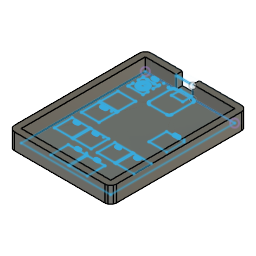
case housing (Autodesk Fusion 360 design; units mm, degrees)
part number: 2026-08-13-11-53-39-217
Autodesk Fusion 360 part; units mm, degrees
(part 1 of 10)
sketch "controller-Edge_Cuts" plane through (0, 0, 3) normal (0, 0, 1) x (1, 0, 0)
  line L0 (34.5096, 49.5231) -> (34.5231, 49.5096)
  line L1 (34.5231, 49.5096) -> (34.525, 49.5)
  line L2 (34.525, 49.5) -> (34.525, -49)
  line L3 (34.525, -49) -> (34.5231, -49.0096)
  line L4 (34.5231, -49.0096) -> (34.5096, -49.0231)
  line L5 (34.5096, -49.0231) -> (34.5, -49.025)
  line L6 (34.5, -49.025) -> (-36.5, -49.025)
  line L7 (-36.5, -49.025) -> (-36.5096, -49.0231)
  line L8 (-36.5096, -49.0231) -> (-36.5231, -49.0096)
  line L9 (-36.5231, -49.0096) -> (-36.525, -49)
  line L10 (-36.525, -49) -> (-36.525, 49.5)
  line L11 (-36.525, 49.5) -> (-36.5231, 49.5096)
  line L12 (-36.5231, 49.5096) -> (-36.5096, 49.5231)
  line L13 (-36.5096, 49.5231) -> (-36.5, 49.525)
  line L14 (-36.5, 49.525) -> (34.5, 49.525)
  line L15 (34.5, 49.525) -> (34.5096, 49.5231)
  line L16 (-36.475, 49.475) -> (-36.475, -48.975)
  line L17 (-36.475, -48.975) -> (34.475, -48.975)
  line L18 (34.475, -48.975) -> (34.475, 49.475)
  line L19 (34.475, 49.475) -> (-36.475, 49.475)
  line L20 (-41.1311, 51.9726) -> (-38.9726, 54.1311)
  line L21 (-38.9726, 54.1311) -> (-36.9925, 54.525)
  line L22 (-36.9925, 54.525) -> (34.9925, 54.525)
  line L23 (34.9925, 54.525) -> (36.9726, 54.1311)
  line L24 (36.9726, 54.1311) -> (39.1311, 51.9726)
  line L25 (39.1311, 51.9726) -> (39.525, 49.9925)
  line L26 (39.525, 49.9925) -> (39.525, -49.4925)
  line L27 (39.525, -49.4925) -> (39.1311, -51.4726)
  line L28 (39.1311, -51.4726) -> (36.9726, -53.6311)
  line L29 (36.9726, -53.6311) -> (34.9925, -54.025)
  line L30 (34.9925, -54.025) -> (-36.9925, -54.025)
  line L31 (-36.9925, -54.025) -> (-38.9726, -53.6311)
  line L32 (-38.9726, -53.6311) -> (-41.1311, -51.4726)
  line L33 (-41.1311, -51.4726) -> (-41.525, -49.4925)
  line L34 (-41.525, -49.4925) -> (-41.525, 49.9925)
  line L35 (-41.525, 49.9925) -> (-41.1311, 51.9726)
  dimension "d53" = -5
extrude "Extrude15" add sketch "controller-Edge_Cuts" along normal blind 3 contours L16 L17 L18 L19 makes body 1
extrude "Extrude16" add sketch "controller-Edge_Cuts" along normal blind 13 separate body contours L20 L21 L22 L23 L24 L25 L26 L27 L28 L29 L30 L31 L32 L33 L34 L35 makes body 2
sketch "controller-F_Silkscreen" plane through (0, 0, 6) normal (0, 0, 1) x (1, 0, 0)
  line L0 (-2.662, -31.4596) -> (-2.6296, -31.492)
  line L1 (-2.6296, -31.492) -> (-2.625, -31.515)
  line L2 (-2.625, -31.515) -> (-2.625, -45.485)
  line L3 (-2.625, -45.485) -> (-2.6296, -45.508)
  line L4 (-2.6296, -45.508) -> (-2.662, -45.5404)
  line L5 (-2.662, -45.5404) -> (-2.685, -45.545)
  line L6 (-2.685, -45.545) -> (-16.655, -45.545)
  line L7 (-16.655, -45.545) -> (-16.678, -45.5404)
  line L8 (-16.678, -45.5404) -> (-16.7104, -45.508)
  line L9 (-16.7104, -45.508) -> (-16.715, -45.485)
  line L10 (-16.715, -45.485) -> (-16.715, -31.515)
  line L11 (-16.715, -31.515) -> (-16.7104, -31.492)
  line L12 (-16.7104, -31.492) -> (-16.678, -31.4596)
  line L13 (-16.678, -31.4596) -> (-16.655, -31.455)
  line L14 (-16.655, -31.455) -> (-2.685, -31.455)
  line L15 (-2.685, -31.455) -> (-2.662, -31.4596)
  line L16 (-16.595, -31.575) -> (-16.595, -45.425)
  line L17 (-16.595, -45.425) -> (-2.745, -45.425)
  line L18 (-2.745, -45.425) -> (-2.745, -31.575)
  line L19 (-2.745, -31.575) -> (-16.595, -31.575)
  line L20 (12.428, -31.4596) -> (12.4604, -31.492)
  line L21 (12.4604, -31.492) -> (12.465, -31.515)
  line L22 (12.465, -31.515) -> (12.465, -45.485)
  line L23 (12.465, -45.485) -> (12.4604, -45.508)
  line L24 (12.4604, -45.508) -> (12.428, -45.5404)
  line L25 (12.428, -45.5404) -> (12.405, -45.545)
  line L26 (12.405, -45.545) -> (-1.565, -45.545)
  line L27 (-1.565, -45.545) -> (-1.588, -45.5404)
  line L28 (-1.588, -45.5404) -> (-1.6204, -45.508)
  line L29 (-1.6204, -45.508) -> (-1.625, -45.485)
  line L30 (-1.625, -45.485) -> (-1.625, -31.515)
  line L31 (-1.625, -31.515) -> (-1.6204, -31.492)
  line L32 (-1.6204, -31.492) -> (-1.588, -31.4596)
  line L33 (-1.588, -31.4596) -> (-1.565, -31.455)
  line L34 (-1.565, -31.455) -> (12.405, -31.455)
  line L35 (12.405, -31.455) -> (12.428, -31.4596)
  line L36 (-1.505, -31.575) -> (-1.505, -45.425)
  line L37 (-1.505, -45.425) -> (12.345, -45.425)
  line L38 (12.345, -45.425) -> (12.345, -31.575)
  line L39 (12.345, -31.575) -> (-1.505, -31.575)
  line L40 (-10.5674, -30.0065) -> (-10.5654, -30.0064)
  line L41 (-10.5654, -30.0064) -> (-10.5628, -30.007)
  line L42 (-10.5628, -30.007) -> (-10.5601, -30.0073)
  line L43 (-10.5601, -30.0073) -> (-10.5583, -30.008)
  line L44 (-10.5583, -30.008) -> (-10.551, -30.0097)
  line L45 (-10.551, -30.0097) -> (-10.4082, -30.0573)
  line L46 (-10.4082, -30.0573) -> (-10.3948, -30.0633)
  line L47 (-10.3948, -30.0633) -> (-10.3727, -30.0825)
  line L48 (-10.3727, -30.0825) -> (-10.3596, -30.1086)
  line L49 (-10.3596, -30.1086) -> (-10.3575, -30.1378)
  line L50 (-10.3575, -30.1378) -> (-10.3667, -30.1656)
  line L51 (-10.3667, -30.1656) -> (-10.3859, -30.1877)
  line L52 (-10.3859, -30.1877) -> (-10.4121, -30.2008)
  line L53 (-10.4121, -30.2008) -> (-10.4413, -30.2028)
  line L54 (-10.4413, -30.2028) -> (-10.4556, -30.1996)
  line L55 (-10.4556, -30.1996) -> (-10.5869, -30.1558)
  line L56 (-10.5869, -30.1558) -> (-10.7952, -30.1558)
  line L57 (-10.7952, -30.1558) -> (-10.8637, -30.1901)
  line L58 (-10.8637, -30.1901) -> (-10.8941, -30.2205)
  line L59 (-10.8941, -30.2205) -> (-10.9283, -30.289)
  line L60 (-10.9283, -30.289) -> (-10.9283, -30.3488)
  line L61 (-10.9283, -30.3488) -> (-10.8941, -30.4173)
  line L62 (-10.8941, -30.4173) -> (-10.8637, -30.4478)
  line L63 (-10.8637, -30.4478) -> (-10.7867, -30.4862)
  line L64 (-10.7867, -30.4862) -> (-10.6042, -30.5319)
  line L65 (-10.6042, -30.5319) -> (-10.6031, -30.5323)
  line L66 (-10.6031, -30.5323) -> (-10.6026, -30.5323)
  line L67 (-10.6026, -30.5323) -> (-10.5965, -30.5346)
  line L68 (-10.5965, -30.5346) -> (-10.5903, -30.5368)
  line L69 (-10.5903, -30.5368) -> (-10.5899, -30.5371)
  line L70 (-10.5899, -30.5371) -> (-10.5888, -30.5375)
  line L71 (-10.5888, -30.5375) -> (-10.4936, -30.5852)
  line L72 (-10.4936, -30.5852) -> (-10.4873, -30.5891)
  line L73 (-10.4873, -30.5891) -> (-10.4855, -30.5899)
  line L74 (-10.4855, -30.5899) -> (-10.4834, -30.5916)
  line L75 (-10.4834, -30.5916) -> (-10.4812, -30.593)
  line L76 (-10.4812, -30.593) -> (-10.4799, -30.5945)
  line L77 (-10.4799, -30.5945) -> (-10.4741, -30.5992)
  line L78 (-10.4741, -30.5992) -> (-10.4265, -30.6468)
  line L79 (-10.4265, -30.6468) -> (-10.4218, -30.6526)
  line L80 (-10.4218, -30.6526) -> (-10.4203, -30.6539)
  line L81 (-10.4203, -30.6539) -> (-10.4189, -30.6561)
  line L82 (-10.4189, -30.6561) -> (-10.4172, -30.6582)
  line L83 (-10.4172, -30.6582) -> (-10.4164, -30.66)
  line L84 (-10.4164, -30.66) -> (-10.4124, -30.6663)
  line L85 (-10.4124, -30.6663) -> (-10.3648, -30.7616)
  line L86 (-10.3648, -30.7616) -> (-10.3596, -30.7753)
  line L87 (-10.3596, -30.7753) -> (-10.3594, -30.778)
  line L88 (-10.3594, -30.778) -> (-10.3583, -30.7805)
  line L89 (-10.3583, -30.7805) -> (-10.3569, -30.7951)
  line L90 (-10.3569, -30.7951) -> (-10.3569, -30.8903)
  line L91 (-10.3569, -30.8903) -> (-10.3583, -30.905)
  line L92 (-10.3583, -30.905) -> (-10.3594, -30.9075)
  line L93 (-10.3594, -30.9075) -> (-10.3596, -30.9102)
  line L94 (-10.3596, -30.9102) -> (-10.3648, -30.9239)
  line L95 (-10.3648, -30.9239) -> (-10.4124, -31.0191)
  line L96 (-10.4124, -31.0191) -> (-10.4164, -31.0254)
  line L97 (-10.4164, -31.0254) -> (-10.4172, -31.0272)
  line L98 (-10.4172, -31.0272) -> (-10.4189, -31.0293)
  line L99 (-10.4189, -31.0293) -> (-10.4203, -31.0316)
  line L100 (-10.4203, -31.0316) -> (-10.4218, -31.0329)
  line L101 (-10.4218, -31.0329) -> (-10.4265, -31.0386)
  line L102 (-10.4265, -31.0386) -> (-10.4741, -31.0862)
  line L103 (-10.4741, -31.0862) -> (-10.4799, -31.0909)
  line L104 (-10.4799, -31.0909) -> (-10.4812, -31.0924)
  line L105 (-10.4812, -31.0924) -> (-10.4834, -31.0939)
  line L106 (-10.4834, -31.0939) -> (-10.4855, -31.0956)
  line L107 (-10.4855, -31.0956) -> (-10.4873, -31.0963)
  line L108 (-10.4873, -31.0963) -> (-10.4936, -31.1003)
  line L109 (-10.4936, -31.1003) -> (-10.5888, -31.1479)
  line L110 (-10.5888, -31.1479) -> (-10.6026, -31.1532)
  line L111 (-10.6026, -31.1532) -> (-10.6053, -31.1533)
  line L112 (-10.6053, -31.1533) -> (-10.6077, -31.1544)
  line L113 (-10.6077, -31.1544) -> (-10.6224, -31.1558)
  line L114 (-10.6224, -31.1558) -> (-10.8605, -31.1558)
  line L115 (-10.8605, -31.1558) -> (-10.8679, -31.1551)
  line L116 (-10.8679, -31.1551) -> (-10.8699, -31.1552)
  line L117 (-10.8699, -31.1552) -> (-10.8725, -31.1546)
  line L118 (-10.8725, -31.1546) -> (-10.8751, -31.1544)
  line L119 (-10.8751, -31.1544) -> (-10.8769, -31.1536)
  line L120 (-10.8769, -31.1536) -> (-10.8842, -31.152)
  line L121 (-10.8842, -31.152) -> (-11.0271, -31.1044)
  line L122 (-11.0271, -31.1044) -> (-11.0405, -31.0984)
  line L123 (-11.0405, -31.0984) -> (-11.0626, -31.0792)
  line L124 (-11.0626, -31.0792) -> (-11.0757, -31.053)
  line L125 (-11.0757, -31.053) -> (-11.0777, -31.0238)
  line L126 (-11.0777, -31.0238) -> (-11.0685, -30.9961)
  line L127 (-11.0685, -30.9961) -> (-11.0493, -30.974)
  line L128 (-11.0493, -30.974) -> (-11.0231, -30.9609)
  line L129 (-11.0231, -30.9609) -> (-10.994, -30.9588)
  line L130 (-10.994, -30.9588) -> (-10.9796, -30.962)
  line L131 (-10.9796, -30.962) -> (-10.8483, -31.0058)
  line L132 (-10.8483, -31.0058) -> (-10.6401, -31.0058)
  line L133 (-10.6401, -31.0058) -> (-10.5716, -30.9716)
  line L134 (-10.5716, -30.9716) -> (-10.5412, -30.9412)
  line L135 (-10.5412, -30.9412) -> (-10.5069, -30.8726)
  line L136 (-10.5069, -30.8726) -> (-10.5069, -30.8128)
  line L137 (-10.5069, -30.8128) -> (-10.5412, -30.7443)
  line L138 (-10.5412, -30.7443) -> (-10.5716, -30.7139)
  line L139 (-10.5716, -30.7139) -> (-10.6486, -30.6754)
  line L140 (-10.6486, -30.6754) -> (-10.831, -30.6298)
  line L141 (-10.831, -30.6298) -> (-10.8321, -30.6294)
  line L142 (-10.8321, -30.6294) -> (-10.8327, -30.6293)
  line L143 (-10.8327, -30.6293) -> (-10.8388, -30.627)
  line L144 (-10.8388, -30.627) -> (-10.8449, -30.6248)
  line L145 (-10.8449, -30.6248) -> (-10.8453, -30.6245)
  line L146 (-10.8453, -30.6245) -> (-10.8464, -30.6241)
  line L147 (-10.8464, -30.6241) -> (-10.9416, -30.5765)
  line L148 (-10.9416, -30.5765) -> (-10.9479, -30.5725)
  line L149 (-10.9479, -30.5725) -> (-10.9498, -30.5717)
  line L150 (-10.9498, -30.5717) -> (-10.9518, -30.5701)
  line L151 (-10.9518, -30.5701) -> (-10.9541, -30.5686)
  line L152 (-10.9541, -30.5686) -> (-10.9554, -30.5671)
  line L153 (-10.9554, -30.5671) -> (-10.9611, -30.5624)
  line L154 (-10.9611, -30.5624) -> (-11.0087, -30.5148)
  line L155 (-11.0087, -30.5148) -> (-11.0135, -30.5091)
  line L156 (-11.0135, -30.5091) -> (-11.015, -30.5078)
  line L157 (-11.015, -30.5078) -> (-11.0164, -30.5055)
  line L158 (-11.0164, -30.5055) -> (-11.0181, -30.5034)
  line L159 (-11.0181, -30.5034) -> (-11.0188, -30.5016)
  line L160 (-11.0188, -30.5016) -> (-11.0228, -30.4953)
  line L161 (-11.0228, -30.4953) -> (-11.0704, -30.4001)
  line L162 (-11.0704, -30.4001) -> (-11.0757, -30.3863)
  line L163 (-11.0757, -30.3863) -> (-11.0759, -30.3837)
  line L164 (-11.0759, -30.3837) -> (-11.0769, -30.3812)
  line L165 (-11.0769, -30.3812) -> (-11.0783, -30.3665)
  line L166 (-11.0783, -30.3665) -> (-11.0783, -30.2713)
  line L167 (-11.0783, -30.2713) -> (-11.0769, -30.2567)
  line L168 (-11.0769, -30.2567) -> (-11.0759, -30.2542)
  line L169 (-11.0759, -30.2542) -> (-11.0757, -30.2515)
  line L170 (-11.0757, -30.2515) -> (-11.0704, -30.2378)
  line L171 (-11.0704, -30.2378) -> (-11.0228, -30.1425)
  line L172 (-11.0228, -30.1425) -> (-11.0188, -30.1362)
  line L173 (-11.0188, -30.1362) -> (-11.0181, -30.1344)
  line L174 (-11.0181, -30.1344) -> (-11.0164, -30.1323)
  line L175 (-11.0164, -30.1323) -> (-11.015, -30.1301)
  line L176 (-11.015, -30.1301) -> (-11.0135, -30.1288)
  line L177 (-11.0135, -30.1288) -> (-11.0087, -30.123)
  line L178 (-11.0087, -30.123) -> (-10.9611, -30.0754)
  line L179 (-10.9611, -30.0754) -> (-10.9554, -30.0707)
  line L180 (-10.9554, -30.0707) -> (-10.9541, -30.0692)
  line L181 (-10.9541, -30.0692) -> (-10.9518, -30.0678)
  line L182 (-10.9518, -30.0678) -> (-10.9498, -30.0661)
  line L183 (-10.9498, -30.0661) -> (-10.9479, -30.0653)
  line L184 (-10.9479, -30.0653) -> (-10.9416, -30.0614)
  line L185 (-10.9416, -30.0614) -> (-10.8464, -30.0137)
  line L186 (-10.8464, -30.0137) -> (-10.8327, -30.0085)
  line L187 (-10.8327, -30.0085) -> (-10.83, -30.0083)
  line L188 (-10.83, -30.0083) -> (-10.8275, -30.0073)
  line L189 (-10.8275, -30.0073) -> (-10.8129, -30.0058)
  line L190 (-10.8129, -30.0058) -> (-10.5748, -30.0058)
  line L191 (-10.5748, -30.0058) -> (-10.5674, -30.0065)
  line L192 (-8.6152, -30.0073) -> (-8.6077, -30.0073)
  line L193 (-8.6077, -30.0073) -> (-8.601, -30.0101)
  line L194 (-8.601, -30.0101) -> (-8.5938, -30.0115)
  line L195 (-8.5938, -30.0115) -> (-8.5876, -30.0156)
  line L196 (-8.5876, -30.0156) -> (-8.5807, -30.0185)
  line L197 (-8.5807, -30.0185) -> (-8.5755, -30.0237)
  line L198 (-8.5755, -30.0237) -> (-8.5694, -30.0277)
  line L199 (-8.5694, -30.0277) -> (-8.5653, -30.0339)
  line L200 (-8.5653, -30.0339) -> (-8.56, -30.0392)
  line L201 (-8.56, -30.0392) -> (-8.5572, -30.0459)
  line L202 (-8.5572, -30.0459) -> (-8.5531, -30.052)
  line L203 (-8.5531, -30.052) -> (-8.5517, -30.0593)
  line L204 (-8.5517, -30.0593) -> (-8.5488, -30.0662)
  line L205 (-8.5488, -30.0662) -> (-8.5474, -30.0807)
  line L206 (-8.5474, -30.0807) -> (-8.5474, -30.0807)
  line L207 (-8.5474, -30.0807) -> (-8.5474, -30.0808)
  line L208 (-8.5474, -30.0808) -> (-8.5474, -30.0808)
  line L209 (-8.5474, -30.0808) -> (-8.5474, -31.0058)
  line L210 (-8.5474, -31.0058) -> (-8.3367, -31.0058)
  line L211 (-8.3367, -31.0058) -> (-8.322, -31.0073)
  line L212 (-8.322, -31.0073) -> (-8.295, -31.0185)
  line L213 (-8.295, -31.0185) -> (-8.2743, -31.0392)
  line L214 (-8.2743, -31.0392) -> (-8.2631, -31.0662)
  line L215 (-8.2631, -31.0662) -> (-8.2631, -31.0955)
  line L216 (-8.2631, -31.0955) -> (-8.2743, -31.1225)
  line L217 (-8.2743, -31.1225) -> (-8.295, -31.1432)
  line L218 (-8.295, -31.1432) -> (-8.322, -31.1544)
  line L219 (-8.322, -31.1544) -> (-8.3367, -31.1558)
  line L220 (-8.3367, -31.1558) -> (-8.9081, -31.1558)
  line L221 (-8.9081, -31.1558) -> (-8.9227, -31.1544)
  line L222 (-8.9227, -31.1544) -> (-8.9498, -31.1432)
  line L223 (-8.9498, -31.1432) -> (-8.9705, -31.1225)
  line L224 (-8.9705, -31.1225) -> (-8.9817, -31.0955)
  line L225 (-8.9817, -31.0955) -> (-8.9817, -31.0662)
  line L226 (-8.9817, -31.0662) -> (-8.9705, -31.0392)
  line L227 (-8.9705, -31.0392) -> (-8.9498, -31.0185)
  line L228 (-8.9498, -31.0185) -> (-8.9227, -31.0073)
  line L229 (-8.9227, -31.0073) -> (-8.9081, -31.0058)
  line L230 (-8.9081, -31.0058) -> (-8.6974, -31.0058)
  line L231 (-8.6974, -31.0058) -> (-8.6974, -30.3095)
  line L232 (-8.6974, -30.3095) -> (-8.7598, -30.3719)
  line L233 (-8.7598, -30.3719) -> (-8.7656, -30.3767)
  line L234 (-8.7656, -30.3767) -> (-8.7669, -30.3782)
  line L235 (-8.7669, -30.3782) -> (-8.7691, -30.3796)
  line L236 (-8.7691, -30.3796) -> (-8.7712, -30.3813)
  line L237 (-8.7712, -30.3813) -> (-8.773, -30.382)
  line L238 (-8.773, -30.382) -> (-8.7793, -30.386)
  line L239 (-8.7793, -30.386) -> (-8.8746, -30.4336)
  line L240 (-8.8746, -30.4336) -> (-8.8883, -30.4389)
  line L241 (-8.8883, -30.4389) -> (-8.9175, -30.4409)
  line L242 (-8.9175, -30.4409) -> (-8.9452, -30.4317)
  line L243 (-8.9452, -30.4317) -> (-8.9673, -30.4125)
  line L244 (-8.9673, -30.4125) -> (-8.9804, -30.3863)
  line L245 (-8.9804, -30.3863) -> (-8.9825, -30.3572)
  line L246 (-8.9825, -30.3572) -> (-8.9733, -30.3294)
  line L247 (-8.9733, -30.3294) -> (-8.9541, -30.3073)
  line L248 (-8.9541, -30.3073) -> (-8.9416, -30.2995)
  line L249 (-8.9416, -30.2995) -> (-8.8573, -30.2573)
  line L250 (-8.8573, -30.2573) -> (-8.7759, -30.1759)
  line L251 (-8.7759, -30.1759) -> (-8.6848, -30.0392)
  line L252 (-8.6848, -30.0392) -> (-8.6848, -30.0392)
  line L253 (-8.6848, -30.0392) -> (-8.6847, -30.0392)
  line L254 (-8.6847, -30.0392) -> (-8.6847, -30.0391)
  line L255 (-8.6847, -30.0391) -> (-8.6755, -30.0278)
  line L256 (-8.6755, -30.0278) -> (-8.6693, -30.0237)
  line L257 (-8.6693, -30.0237) -> (-8.664, -30.0185)
  line L258 (-8.664, -30.0185) -> (-8.6573, -30.0156)
  line L259 (-8.6573, -30.0156) -> (-8.6512, -30.0116)
  line L260 (-8.6512, -30.0116) -> (-8.6439, -30.0101)
  line L261 (-8.6439, -30.0101) -> (-8.637, -30.0073)
  line L262 (-8.637, -30.0073) -> (-8.6297, -30.0073)
  line L263 (-8.6297, -30.0073) -> (-8.6225, -30.0058)
  line L264 (-8.6225, -30.0058) -> (-8.6152, -30.0073)
  line L265 (4.5226, -30.0065) -> (4.5246, -30.0064)
  line L266 (4.5246, -30.0064) -> (4.5272, -30.007)
  line L267 (4.5272, -30.007) -> (4.5299, -30.0073)
  line L268 (4.5299, -30.0073) -> (4.5317, -30.008)
  line L269 (4.5317, -30.008) -> (4.539, -30.0097)
  line L270 (4.539, -30.0097) -> (4.6818, -30.0573)
  line L271 (4.6818, -30.0573) -> (4.6952, -30.0633)
  line L272 (4.6952, -30.0633) -> (4.7173, -30.0825)
  line L273 (4.7173, -30.0825) -> (4.7304, -30.1086)
  line L274 (4.7304, -30.1086) -> (4.7325, -30.1378)
  line L275 (4.7325, -30.1378) -> (4.7233, -30.1656)
  line L276 (4.7233, -30.1656) -> (4.7041, -30.1877)
  line L277 (4.7041, -30.1877) -> (4.6779, -30.2008)
  line L278 (4.6779, -30.2008) -> (4.6487, -30.2028)
  line L279 (4.6487, -30.2028) -> (4.6344, -30.1996)
  line L280 (4.6344, -30.1996) -> (4.5031, -30.1558)
  line L281 (4.5031, -30.1558) -> (4.2948, -30.1558)
  line L282 (4.2948, -30.1558) -> (4.2263, -30.1901)
  line L283 (4.2263, -30.1901) -> (4.1959, -30.2205)
  line L284 (4.1959, -30.2205) -> (4.1617, -30.289)
  line L285 (4.1617, -30.289) -> (4.1617, -30.3488)
  line L286 (4.1617, -30.3488) -> (4.1959, -30.4173)
  line L287 (4.1959, -30.4173) -> (4.2263, -30.4478)
  line L288 (4.2263, -30.4478) -> (4.3033, -30.4862)
  line L289 (4.3033, -30.4862) -> (4.4858, -30.5319)
  line L290 (4.4858, -30.5319) -> (4.4869, -30.5323)
  line L291 (4.4869, -30.5323) -> (4.4874, -30.5323)
  line L292 (4.4874, -30.5323) -> (4.4935, -30.5346)
  line L293 (4.4935, -30.5346) -> (4.4997, -30.5368)
  line L294 (4.4997, -30.5368) -> (4.5001, -30.5371)
  line L295 (4.5001, -30.5371) -> (4.5012, -30.5375)
  line L296 (4.5012, -30.5375) -> (4.5964, -30.5852)
  line L297 (4.5964, -30.5852) -> (4.6027, -30.5891)
  line L298 (4.6027, -30.5891) -> (4.6045, -30.5899)
  line L299 (4.6045, -30.5899) -> (4.6066, -30.5916)
  line L300 (4.6066, -30.5916) -> (4.6088, -30.593)
  line L301 (4.6088, -30.593) -> (4.6101, -30.5945)
  line L302 (4.6101, -30.5945) -> (4.6159, -30.5992)
  line L303 (4.6159, -30.5992) -> (4.6635, -30.6468)
  line L304 (4.6635, -30.6468) -> (4.6682, -30.6526)
  line L305 (4.6682, -30.6526) -> (4.6697, -30.6539)
  line L306 (4.6697, -30.6539) -> (4.6711, -30.6561)
  line L307 (4.6711, -30.6561) -> (4.6728, -30.6582)
  line L308 (4.6728, -30.6582) -> (4.6736, -30.66)
  line L309 (4.6736, -30.66) -> (4.6776, -30.6663)
  line L310 (4.6776, -30.6663) -> (4.7252, -30.7616)
  line L311 (4.7252, -30.7616) -> (4.7304, -30.7753)
  line L312 (4.7304, -30.7753) -> (4.7306, -30.778)
  line L313 (4.7306, -30.778) -> (4.7317, -30.7805)
  line L314 (4.7317, -30.7805) -> (4.7331, -30.7951)
  line L315 (4.7331, -30.7951) -> (4.7331, -30.8903)
  line L316 (4.7331, -30.8903) -> (4.7317, -30.905)
  line L317 (4.7317, -30.905) -> (4.7306, -30.9075)
  line L318 (4.7306, -30.9075) -> (4.7304, -30.9102)
  line L319 (4.7304, -30.9102) -> (4.7252, -30.9239)
  line L320 (4.7252, -30.9239) -> (4.6776, -31.0191)
  line L321 (4.6776, -31.0191) -> (4.6736, -31.0254)
  line L322 (4.6736, -31.0254) -> (4.6728, -31.0272)
  line L323 (4.6728, -31.0272) -> (4.6711, -31.0293)
  line L324 (4.6711, -31.0293) -> (4.6697, -31.0316)
  line L325 (4.6697, -31.0316) -> (4.6682, -31.0329)
  line L326 (4.6682, -31.0329) -> (4.6635, -31.0386)
  line L327 (4.6635, -31.0386) -> (4.6159, -31.0862)
  line L328 (4.6159, -31.0862) -> (4.6101, -31.0909)
  line L329 (4.6101, -31.0909) -> (4.6088, -31.0924)
  line L330 (4.6088, -31.0924) -> (4.6066, -31.0939)
  line L331 (4.6066, -31.0939) -> (4.6045, -31.0956)
  line L332 (4.6045, -31.0956) -> (4.6027, -31.0963)
  line L333 (4.6027, -31.0963) -> (4.5964, -31.1003)
  line L334 (4.5964, -31.1003) -> (4.5012, -31.1479)
  line L335 (4.5012, -31.1479) -> (4.4874, -31.1532)
  line L336 (4.4874, -31.1532) -> (4.4847, -31.1533)
  line L337 (4.4847, -31.1533) -> (4.4823, -31.1544)
  line L338 (4.4823, -31.1544) -> (4.4676, -31.1558)
  line L339 (4.4676, -31.1558) -> (4.2295, -31.1558)
  line L340 (4.2295, -31.1558) -> (4.2221, -31.1551)
  line L341 (4.2221, -31.1551) -> (4.2201, -31.1552)
  line L342 (4.2201, -31.1552) -> (4.2175, -31.1546)
  line L343 (4.2175, -31.1546) -> (4.2149, -31.1544)
  line L344 (4.2149, -31.1544) -> (4.2131, -31.1536)
  line L345 (4.2131, -31.1536) -> (4.2058, -31.152)
  line L346 (4.2058, -31.152) -> (4.063, -31.1044)
  line L347 (4.063, -31.1044) -> (4.0495, -31.0984)
  line L348 (4.0495, -31.0984) -> (4.0274, -31.0792)
  line L349 (4.0274, -31.0792) -> (4.0143, -31.053)
  line L350 (4.0143, -31.053) -> (4.0123, -31.0238)
  line L351 (4.0123, -31.0238) -> (4.0215, -30.9961)
  line L352 (4.0215, -30.9961) -> (4.0407, -30.974)
  line L353 (4.0407, -30.974) -> (4.0669, -30.9609)
  line L354 (4.0669, -30.9609) -> (4.096, -30.9588)
  line L355 (4.096, -30.9588) -> (4.1104, -30.962)
  line L356 (4.1104, -30.962) -> (4.2417, -31.0058)
  line L357 (4.2417, -31.0058) -> (4.4499, -31.0058)
  line L358 (4.4499, -31.0058) -> (4.5184, -30.9716)
  line L359 (4.5184, -30.9716) -> (4.5488, -30.9412)
  line L360 (4.5488, -30.9412) -> (4.5831, -30.8726)
  line L361 (4.5831, -30.8726) -> (4.5831, -30.8128)
  line L362 (4.5831, -30.8128) -> (4.5488, -30.7443)
  line L363 (4.5488, -30.7443) -> (4.5184, -30.7139)
  line L364 (4.5184, -30.7139) -> (4.4414, -30.6754)
  line L365 (4.4414, -30.6754) -> (4.259, -30.6298)
  line L366 (4.259, -30.6298) -> (4.2579, -30.6294)
  line L367 (4.2579, -30.6294) -> (4.2573, -30.6293)
  line L368 (4.2573, -30.6293) -> (4.2512, -30.627)
  line L369 (4.2512, -30.627) -> (4.2451, -30.6248)
  line L370 (4.2451, -30.6248) -> (4.2447, -30.6245)
  line L371 (4.2447, -30.6245) -> (4.2436, -30.6241)
  line L372 (4.2436, -30.6241) -> (4.1484, -30.5765)
  line L373 (4.1484, -30.5765) -> (4.1421, -30.5725)
  line L374 (4.1421, -30.5725) -> (4.1402, -30.5717)
  line L375 (4.1402, -30.5717) -> (4.1382, -30.5701)
  line L376 (4.1382, -30.5701) -> (4.1359, -30.5686)
  line L377 (4.1359, -30.5686) -> (4.1346, -30.5671)
  line L378 (4.1346, -30.5671) -> (4.1289, -30.5624)
  line L379 (4.1289, -30.5624) -> (4.0813, -30.5148)
  line L380 (4.0813, -30.5148) -> (4.0765, -30.5091)
  line L381 (4.0765, -30.5091) -> (4.075, -30.5078)
  line L382 (4.075, -30.5078) -> (4.0736, -30.5055)
  line L383 (4.0736, -30.5055) -> (4.0719, -30.5034)
  line L384 (4.0719, -30.5034) -> (4.0712, -30.5016)
  line L385 (4.0712, -30.5016) -> (4.0672, -30.4953)
  line L386 (4.0672, -30.4953) -> (4.0196, -30.4001)
  line L387 (4.0196, -30.4001) -> (4.0143, -30.3863)
  line L388 (4.0143, -30.3863) -> (4.0141, -30.3837)
  line L389 (4.0141, -30.3837) -> (4.0131, -30.3812)
  line L390 (4.0131, -30.3812) -> (4.0117, -30.3665)
  line L391 (4.0117, -30.3665) -> (4.0117, -30.2713)
  line L392 (4.0117, -30.2713) -> (4.0131, -30.2567)
  line L393 (4.0131, -30.2567) -> (4.0141, -30.2542)
  line L394 (4.0141, -30.2542) -> (4.0143, -30.2515)
  line L395 (4.0143, -30.2515) -> (4.0196, -30.2378)
  line L396 (4.0196, -30.2378) -> (4.0672, -30.1425)
  line L397 (4.0672, -30.1425) -> (4.0712, -30.1362)
  line L398 (4.0712, -30.1362) -> (4.0719, -30.1344)
  line L399 (4.0719, -30.1344) -> (4.0736, -30.1323)
  line L400 (4.0736, -30.1323) -> (4.075, -30.1301)
  line L401 (4.075, -30.1301) -> (4.0765, -30.1288)
  line L402 (4.0765, -30.1288) -> (4.0813, -30.123)
  line L403 (4.0813, -30.123) -> (4.1289, -30.0754)
  line L404 (4.1289, -30.0754) -> (4.1346, -30.0707)
  line L405 (4.1346, -30.0707) -> (4.1359, -30.0692)
  line L406 (4.1359, -30.0692) -> (4.1382, -30.0678)
  line L407 (4.1382, -30.0678) -> (4.1402, -30.0661)
  line L408 (4.1402, -30.0661) -> (4.1421, -30.0653)
  line L409 (4.1421, -30.0653) -> (4.1484, -30.0614)
  line L410 (4.1484, -30.0614) -> (4.2436, -30.0137)
  line L411 (4.2436, -30.0137) -> (4.2573, -30.0085)
  line L412 (4.2573, -30.0085) -> (4.26, -30.0083)
  line L413 (4.26, -30.0083) -> (4.2625, -30.0073)
  line L414 (4.2625, -30.0073) -> (4.2771, -30.0058)
  line L415 (4.2771, -30.0058) -> (4.5152, -30.0058)
  line L416 (4.5152, -30.0058) -> (4.5226, -30.0065)
  line L417 (6.7203, -30.0073) -> (6.7474, -30.0185)
  line L418 (6.7474, -30.0185) -> (6.7681, -30.0392)
  line L419 (6.7681, -30.0392) -> (6.7793, -30.0662)
  line L420 (6.7793, -30.0662) -> (6.7793, -30.0955)
  line L421 (6.7793, -30.0955) -> (6.7681, -30.1225)
  line L422 (6.7681, -30.1225) -> (6.7474, -30.1432)
  line L423 (6.7474, -30.1432) -> (6.7203, -30.1544)
  line L424 (6.7203, -30.1544) -> (6.7057, -30.1558)
  line L425 (6.7057, -30.1558) -> (6.2974, -30.1558)
  line L426 (6.2974, -30.1558) -> (6.2726, -30.404)
  line L427 (6.2726, -30.404) -> (6.2912, -30.3947)
  line L428 (6.2912, -30.3947) -> (6.305, -30.3894)
  line L429 (6.305, -30.3894) -> (6.3076, -30.3892)
  line L430 (6.3076, -30.3892) -> (6.3101, -30.3882)
  line L431 (6.3101, -30.3882) -> (6.3248, -30.3868)
  line L432 (6.3248, -30.3868) -> (6.5629, -30.3868)
  line L433 (6.5629, -30.3868) -> (6.5775, -30.3882)
  line L434 (6.5775, -30.3882) -> (6.58, -30.3892)
  line L435 (6.58, -30.3892) -> (6.5827, -30.3894)
  line L436 (6.5827, -30.3894) -> (6.5964, -30.3947)
  line L437 (6.5964, -30.3947) -> (6.6916, -30.4423)
  line L438 (6.6916, -30.4423) -> (6.6979, -30.4463)
  line L439 (6.6979, -30.4463) -> (6.6998, -30.447)
  line L440 (6.6998, -30.447) -> (6.7018, -30.4487)
  line L441 (6.7018, -30.4487) -> (6.7041, -30.4501)
  line L442 (6.7041, -30.4501) -> (6.7054, -30.4516)
  line L443 (6.7054, -30.4516) -> (6.7111, -30.4564)
  line L444 (6.7111, -30.4564) -> (6.7587, -30.504)
  line L445 (6.7587, -30.504) -> (6.7635, -30.5097)
  line L446 (6.7635, -30.5097) -> (6.765, -30.511)
  line L447 (6.765, -30.511) -> (6.7664, -30.5133)
  line L448 (6.7664, -30.5133) -> (6.7681, -30.5153)
  line L449 (6.7681, -30.5153) -> (6.7688, -30.5172)
  line L450 (6.7688, -30.5172) -> (6.7728, -30.5235)
  line L451 (6.7728, -30.5235) -> (6.8204, -30.6187)
  line L452 (6.8204, -30.6187) -> (6.8257, -30.6324)
  line L453 (6.8257, -30.6324) -> (6.8259, -30.6351)
  line L454 (6.8259, -30.6351) -> (6.8269, -30.6376)
  line L455 (6.8269, -30.6376) -> (6.8283, -30.6522)
  line L456 (6.8283, -30.6522) -> (6.8283, -30.8903)
  line L457 (6.8283, -30.8903) -> (6.8269, -30.905)
  line L458 (6.8269, -30.905) -> (6.8259, -30.9075)
  line L459 (6.8259, -30.9075) -> (6.8257, -30.9102)
  line L460 (6.8257, -30.9102) -> (6.8204, -30.9239)
  line L461 (6.8204, -30.9239) -> (6.7728, -31.0191)
  line L462 (6.7728, -31.0191) -> (6.7688, -31.0254)
  line L463 (6.7688, -31.0254) -> (6.7681, -31.0272)
  line L464 (6.7681, -31.0272) -> (6.7664, -31.0293)
  line L465 (6.7664, -31.0293) -> (6.765, -31.0316)
  line L466 (6.765, -31.0316) -> (6.7635, -31.0329)
  line L467 (6.7635, -31.0329) -> (6.7587, -31.0386)
  line L468 (6.7587, -31.0386) -> (6.7111, -31.0862)
  line L469 (6.7111, -31.0862) -> (6.7054, -31.0909)
  line L470 (6.7054, -31.0909) -> (6.7041, -31.0924)
  line L471 (6.7041, -31.0924) -> (6.7018, -31.0939)
  line L472 (6.7018, -31.0939) -> (6.6998, -31.0956)
  line L473 (6.6998, -31.0956) -> (6.6979, -31.0963)
  line L474 (6.6979, -31.0963) -> (6.6916, -31.1003)
  line L475 (6.6916, -31.1003) -> (6.5964, -31.1479)
  line L476 (6.5964, -31.1479) -> (6.5827, -31.1532)
  line L477 (6.5827, -31.1532) -> (6.58, -31.1533)
  line L478 (6.58, -31.1533) -> (6.5775, -31.1544)
  line L479 (6.5775, -31.1544) -> (6.5629, -31.1558)
  line L480 (6.5629, -31.1558) -> (6.3248, -31.1558)
  line L481 (6.3248, -31.1558) -> (6.3101, -31.1544)
  line L482 (6.3101, -31.1544) -> (6.3076, -31.1533)
  line L483 (6.3076, -31.1533) -> (6.305, -31.1532)
  line L484 (6.305, -31.1532) -> (6.2912, -31.1479)
  line L485 (6.2912, -31.1479) -> (6.196, -31.1003)
  line L486 (6.196, -31.1003) -> (6.1897, -31.0963)
  line L487 (6.1897, -31.0963) -> (6.1879, -31.0956)
  line L488 (6.1879, -31.0956) -> (6.1858, -31.0939)
  line L489 (6.1858, -31.0939) -> (6.1835, -31.0924)
  line L490 (6.1835, -31.0924) -> (6.1822, -31.0909)
  line L491 (6.1822, -31.0909) -> (6.1765, -31.0862)
  line L492 (6.1765, -31.0862) -> (6.1289, -31.0386)
  line L493 (6.1289, -31.0386) -> (6.1195, -31.0272)
  line L494 (6.1195, -31.0272) -> (6.1083, -31.0002)
  line L495 (6.1083, -31.0002) -> (6.1083, -30.9709)
  line L496 (6.1083, -30.9709) -> (6.1195, -30.9439)
  line L497 (6.1195, -30.9439) -> (6.1402, -30.9232)
  line L498 (6.1402, -30.9232) -> (6.1673, -30.912)
  line L499 (6.1673, -30.912) -> (6.1965, -30.912)
  line L500 (6.1965, -30.912) -> (6.2236, -30.9232)
  line L501 (6.2236, -30.9232) -> (6.2349, -30.9325)
  line L502 (6.2349, -30.9325) -> (6.274, -30.9716)
  line L503 (6.274, -30.9716) -> (6.3425, -31.0058)
  line L504 (6.3425, -31.0058) -> (6.5452, -31.0058)
  line L505 (6.5452, -31.0058) -> (6.6137, -30.9716)
  line L506 (6.6137, -30.9716) -> (6.6441, -30.9412)
  line L507 (6.6441, -30.9412) -> (6.6783, -30.8726)
  line L508 (6.6783, -30.8726) -> (6.6783, -30.67)
  line L509 (6.6783, -30.67) -> (6.6441, -30.6014)
  line L510 (6.6441, -30.6014) -> (6.6137, -30.571)
  line L511 (6.6137, -30.571) -> (6.5452, -30.5368)
  line L512 (6.5452, -30.5368) -> (6.3425, -30.5368)
  line L513 (6.3425, -30.5368) -> (6.274, -30.571)
  line L514 (6.274, -30.571) -> (6.2349, -30.61)
  line L515 (6.2349, -30.61) -> (6.2236, -30.6194)
  line L516 (6.2236, -30.6194) -> (6.2201, -30.6208)
  line L517 (6.2201, -30.6208) -> (6.2172, -30.6232)
  line L518 (6.2172, -30.6232) -> (6.2067, -30.6264)
  line L519 (6.2067, -30.6264) -> (6.1965, -30.6306)
  line L520 (6.1965, -30.6306) -> (6.1928, -30.6306)
  line L521 (6.1928, -30.6306) -> (6.1891, -30.6317)
  line L522 (6.1891, -30.6317) -> (6.1782, -30.6306)
  line L523 (6.1782, -30.6306) -> (6.1673, -30.6306)
  line L524 (6.1673, -30.6306) -> (6.1638, -30.6291)
  line L525 (6.1638, -30.6291) -> (6.16, -30.6287)
  line L526 (6.16, -30.6287) -> (6.1504, -30.6236)
  line L527 (6.1504, -30.6236) -> (6.1402, -30.6194)
  line L528 (6.1402, -30.6194) -> (6.1376, -30.6167)
  line L529 (6.1376, -30.6167) -> (6.1342, -30.6149)
  line L530 (6.1342, -30.6149) -> (6.1273, -30.6064)
  line L531 (6.1273, -30.6064) -> (6.1195, -30.5987)
  line L532 (6.1195, -30.5987) -> (6.1181, -30.5952)
  line L533 (6.1181, -30.5952) -> (6.1157, -30.5923)
  line L534 (6.1157, -30.5923) -> (6.1125, -30.5818)
  line L535 (6.1125, -30.5818) -> (6.1083, -30.5716)
  line L536 (6.1083, -30.5716) -> (6.1083, -30.5679)
  line L537 (6.1083, -30.5679) -> (6.1073, -30.5642)
  line L538 (6.1073, -30.5642) -> (6.1073, -30.5495)
  line L539 (6.1073, -30.5495) -> (6.1549, -30.0734)
  line L540 (6.1549, -30.0734) -> (6.156, -30.068)
  line L541 (6.156, -30.068) -> (6.156, -30.0662)
  line L542 (6.156, -30.0662) -> (6.1567, -30.0645)
  line L543 (6.1567, -30.0645) -> (6.1578, -30.0589)
  line L544 (6.1578, -30.0589) -> (6.163, -30.0493)
  line L545 (6.163, -30.0493) -> (6.1672, -30.0392)
  line L546 (6.1672, -30.0392) -> (6.1698, -30.0365)
  line L547 (6.1698, -30.0365) -> (6.1716, -30.0332)
  line L548 (6.1716, -30.0332) -> (6.1801, -30.0262)
  line L549 (6.1801, -30.0262) -> (6.1879, -30.0185)
  line L550 (6.1879, -30.0185) -> (6.1913, -30.017)
  line L551 (6.1913, -30.017) -> (6.1943, -30.0146)
  line L552 (6.1943, -30.0146) -> (6.2048, -30.0115)
  line L553 (6.2048, -30.0115) -> (6.2149, -30.0073)
  line L554 (6.2149, -30.0073) -> (6.2205, -30.0067)
  line L555 (6.2205, -30.0067) -> (6.2223, -30.0062)
  line L556 (6.2223, -30.0062) -> (6.2241, -30.0064)
  line L557 (6.2241, -30.0064) -> (6.2295, -30.0058)
  line L558 (6.2295, -30.0058) -> (6.7057, -30.0058)
  line L559 (6.7057, -30.0058) -> (6.7203, -30.0073)
  line L560 (-9.2102, -30.0127) -> (-9.1864, -30.0298)
  line L561 (-9.1864, -30.0298) -> (-9.1711, -30.0547)
  line L562 (-9.1711, -30.0547) -> (-9.1665, -30.0836)
  line L563 (-9.1665, -30.0836) -> (-9.1685, -30.0982)
  line L564 (-9.1685, -30.0982) -> (-9.4066, -31.0982)
  line L565 (-9.4066, -31.0982) -> (-9.4083, -31.1032)
  line L566 (-9.4083, -31.1032) -> (-9.4085, -31.105)
  line L567 (-9.4085, -31.105) -> (-9.4095, -31.1066)
  line L568 (-9.4095, -31.1066) -> (-9.4114, -31.1121)
  line L569 (-9.4114, -31.1121) -> (-9.4177, -31.1209)
  line L570 (-9.4177, -31.1209) -> (-9.4232, -31.1303)
  line L571 (-9.4232, -31.1303) -> (-9.4263, -31.1327)
  line L572 (-9.4263, -31.1327) -> (-9.4285, -31.1358)
  line L573 (-9.4285, -31.1358) -> (-9.4378, -31.1415)
  line L574 (-9.4378, -31.1415) -> (-9.4464, -31.1481)
  line L575 (-9.4464, -31.1481) -> (-9.4502, -31.1491)
  line L576 (-9.4502, -31.1491) -> (-9.4534, -31.1511)
  line L577 (-9.4534, -31.1511) -> (-9.4642, -31.1529)
  line L578 (-9.4642, -31.1529) -> (-9.4747, -31.1557)
  line L579 (-9.4747, -31.1557) -> (-9.4785, -31.1552)
  line L580 (-9.4785, -31.1552) -> (-9.4823, -31.1558)
  line L581 (-9.4823, -31.1558) -> (-9.4929, -31.1532)
  line L582 (-9.4929, -31.1532) -> (-9.5037, -31.1518)
  line L583 (-9.5037, -31.1518) -> (-9.507, -31.1499)
  line L584 (-9.507, -31.1499) -> (-9.5108, -31.149)
  line L585 (-9.5108, -31.149) -> (-9.5196, -31.1426)
  line L586 (-9.5196, -31.1426) -> (-9.529, -31.1371)
  line L587 (-9.529, -31.1371) -> (-9.5314, -31.1341)
  line L588 (-9.5314, -31.1341) -> (-9.5345, -31.1318)
  line L589 (-9.5345, -31.1318) -> (-9.5402, -31.1226)
  line L590 (-9.5402, -31.1226) -> (-9.5468, -31.1139)
  line L591 (-9.5468, -31.1139) -> (-9.5489, -31.1085)
  line L592 (-9.5489, -31.1085) -> (-9.5498, -31.1069)
  line L593 (-9.5498, -31.1069) -> (-9.5501, -31.1051)
  line L594 (-9.5501, -31.1051) -> (-9.552, -31.1001)
  line L595 (-9.552, -31.1001) -> (-9.67, -30.6576)
  line L596 (-9.67, -30.6576) -> (-9.788, -31.1001)
  line L597 (-9.788, -31.1001) -> (-9.7899, -31.1051)
  line L598 (-9.7899, -31.1051) -> (-9.7902, -31.1069)
  line L599 (-9.7902, -31.1069) -> (-9.7911, -31.1085)
  line L600 (-9.7911, -31.1085) -> (-9.7932, -31.1139)
  line L601 (-9.7932, -31.1139) -> (-9.7998, -31.1226)
  line L602 (-9.7998, -31.1226) -> (-9.8055, -31.1318)
  line L603 (-9.8055, -31.1318) -> (-9.8086, -31.1341)
  line L604 (-9.8086, -31.1341) -> (-9.811, -31.1371)
  line L605 (-9.811, -31.1371) -> (-9.8204, -31.1426)
  line L606 (-9.8204, -31.1426) -> (-9.8292, -31.149)
  line L607 (-9.8292, -31.149) -> (-9.833, -31.1499)
  line L608 (-9.833, -31.1499) -> (-9.8363, -31.1518)
  line L609 (-9.8363, -31.1518) -> (-9.8471, -31.1532)
  line L610 (-9.8471, -31.1532) -> (-9.8577, -31.1558)
  line L611 (-9.8577, -31.1558) -> (-9.8615, -31.1552)
  line L612 (-9.8615, -31.1552) -> (-9.8653, -31.1557)
  line L613 (-9.8653, -31.1557) -> (-9.8758, -31.1529)
  line L614 (-9.8758, -31.1529) -> (-9.8866, -31.1511)
  line L615 (-9.8866, -31.1511) -> (-9.8898, -31.1491)
  line L616 (-9.8898, -31.1491) -> (-9.8936, -31.1481)
  line L617 (-9.8936, -31.1481) -> (-9.9022, -31.1415)
  line L618 (-9.9022, -31.1415) -> (-9.9115, -31.1358)
  line L619 (-9.9115, -31.1358) -> (-9.9137, -31.1327)
  line L620 (-9.9137, -31.1327) -> (-9.9168, -31.1303)
  line L621 (-9.9168, -31.1303) -> (-9.9223, -31.1209)
  line L622 (-9.9223, -31.1209) -> (-9.9286, -31.1121)
  line L623 (-9.9286, -31.1121) -> (-9.9305, -31.1066)
  line L624 (-9.9305, -31.1066) -> (-9.9315, -31.105)
  line L625 (-9.9315, -31.105) -> (-9.9317, -31.1032)
  line L626 (-9.9317, -31.1032) -> (-9.9334, -31.0982)
  line L627 (-9.9334, -31.0982) -> (-10.1715, -30.0982)
  line L628 (-10.1715, -30.0982) -> (-10.1735, -30.0836)
  line L629 (-10.1735, -30.0836) -> (-10.1689, -30.0547)
  line L630 (-10.1689, -30.0547) -> (-10.1535, -30.0298)
  line L631 (-10.1535, -30.0298) -> (-10.1298, -30.0126)
  line L632 (-10.1298, -30.0126) -> (-10.1014, -30.0059)
  line L633 (-10.1014, -30.0059) -> (-10.0725, -30.0105)
  line L634 (-10.0725, -30.0105) -> (-10.0476, -30.0258)
  line L635 (-10.0476, -30.0258) -> (-10.0304, -30.0495)
  line L636 (-10.0304, -30.0495) -> (-10.0256, -30.0634)
  line L637 (-10.0256, -30.0634) -> (-9.8564, -30.7743)
  line L638 (-9.8564, -30.7743) -> (-9.7425, -30.3472)
  line L639 (-9.7425, -30.3472) -> (-9.7412, -30.3438)
  line L640 (-9.7412, -30.3438) -> (-9.741, -30.3423)
  line L641 (-9.741, -30.3423) -> (-9.74, -30.3406)
  line L642 (-9.74, -30.3406) -> (-9.7373, -30.3334)
  line L643 (-9.7373, -30.3334) -> (-9.7313, -30.3256)
  line L644 (-9.7313, -30.3256) -> (-9.7263, -30.317)
  line L645 (-9.7263, -30.317) -> (-9.7225, -30.3141)
  line L646 (-9.7225, -30.3141) -> (-9.7195, -30.3102)
  line L647 (-9.7195, -30.3102) -> (-9.711, -30.3052)
  line L648 (-9.711, -30.3052) -> (-9.7031, -30.2992)
  line L649 (-9.7031, -30.2992) -> (-9.6984, -30.298)
  line L650 (-9.6984, -30.298) -> (-9.6942, -30.2955)
  line L651 (-9.6942, -30.2955) -> (-9.6844, -30.2942)
  line L652 (-9.6844, -30.2942) -> (-9.6748, -30.2917)
  line L653 (-9.6748, -30.2917) -> (-9.67, -30.2923)
  line L654 (-9.67, -30.2923) -> (-9.6652, -30.2917)
  line L655 (-9.6652, -30.2917) -> (-9.6556, -30.2942)
  line L656 (-9.6556, -30.2942) -> (-9.6458, -30.2955)
  line L657 (-9.6458, -30.2955) -> (-9.6416, -30.298)
  line L658 (-9.6416, -30.298) -> (-9.6369, -30.2992)
  line L659 (-9.6369, -30.2992) -> (-9.629, -30.3052)
  line L660 (-9.629, -30.3052) -> (-9.6205, -30.3102)
  line L661 (-9.6205, -30.3102) -> (-9.6175, -30.3141)
  line L662 (-9.6175, -30.3141) -> (-9.6137, -30.317)
  line L663 (-9.6137, -30.317) -> (-9.6087, -30.3256)
  line L664 (-9.6087, -30.3256) -> (-9.6027, -30.3334)
  line L665 (-9.6027, -30.3334) -> (-9.6, -30.3406)
  line L666 (-9.6, -30.3406) -> (-9.599, -30.3423)
  line L667 (-9.599, -30.3423) -> (-9.5988, -30.3438)
  line L668 (-9.5988, -30.3438) -> (-9.5975, -30.3472)
  line L669 (-9.5975, -30.3472) -> (-9.4836, -30.7743)
  line L670 (-9.4836, -30.7743) -> (-9.3144, -30.0634)
  line L671 (-9.3144, -30.0634) -> (-9.3096, -30.0495)
  line L672 (-9.3096, -30.0495) -> (-9.2924, -30.0258)
  line L673 (-9.2924, -30.0258) -> (-9.2675, -30.0105)
  line L674 (-9.2675, -30.0105) -> (-9.2386, -30.0059)
  line L675 (-9.2386, -30.0059) -> (-9.2102, -30.0127)
  line L676 (5.8798, -30.0127) -> (5.9036, -30.0298)
  line L677 (5.9036, -30.0298) -> (5.9189, -30.0547)
  line L678 (5.9189, -30.0547) -> (5.9235, -30.0836)
  line L679 (5.9235, -30.0836) -> (5.9215, -30.0982)
  line L680 (5.9215, -30.0982) -> (5.6834, -31.0982)
  line L681 (5.6834, -31.0982) -> (5.6817, -31.1032)
  line L682 (5.6817, -31.1032) -> (5.6815, -31.105)
  line L683 (5.6815, -31.105) -> (5.6805, -31.1066)
  line L684 (5.6805, -31.1066) -> (5.6786, -31.1121)
  line L685 (5.6786, -31.1121) -> (5.6723, -31.1209)
  line L686 (5.6723, -31.1209) -> (5.6668, -31.1303)
  line L687 (5.6668, -31.1303) -> (5.6637, -31.1327)
  line L688 (5.6637, -31.1327) -> (5.6615, -31.1358)
  line L689 (5.6615, -31.1358) -> (5.6522, -31.1415)
  line L690 (5.6522, -31.1415) -> (5.6436, -31.1481)
  line L691 (5.6436, -31.1481) -> (5.6398, -31.1491)
  line L692 (5.6398, -31.1491) -> (5.6366, -31.1511)
  line L693 (5.6366, -31.1511) -> (5.6258, -31.1529)
  line L694 (5.6258, -31.1529) -> (5.6153, -31.1557)
  line L695 (5.6153, -31.1557) -> (5.6115, -31.1552)
  line L696 (5.6115, -31.1552) -> (5.6077, -31.1558)
  line L697 (5.6077, -31.1558) -> (5.5971, -31.1532)
  line L698 (5.5971, -31.1532) -> (5.5863, -31.1518)
  line L699 (5.5863, -31.1518) -> (5.583, -31.1499)
  line L700 (5.583, -31.1499) -> (5.5792, -31.149)
  line L701 (5.5792, -31.149) -> (5.5704, -31.1426)
  line L702 (5.5704, -31.1426) -> (5.561, -31.1371)
  line L703 (5.561, -31.1371) -> (5.5586, -31.1341)
  line L704 (5.5586, -31.1341) -> (5.5555, -31.1318)
  line L705 (5.5555, -31.1318) -> (5.5498, -31.1226)
  line L706 (5.5498, -31.1226) -> (5.5432, -31.1139)
  line L707 (5.5432, -31.1139) -> (5.5411, -31.1085)
  line L708 (5.5411, -31.1085) -> (5.5402, -31.1069)
  line L709 (5.5402, -31.1069) -> (5.5399, -31.1051)
  line L710 (5.5399, -31.1051) -> (5.538, -31.1001)
  line L711 (5.538, -31.1001) -> (5.42, -30.6576)
  line L712 (5.42, -30.6576) -> (5.302, -31.1001)
  line L713 (5.302, -31.1001) -> (5.3001, -31.1051)
  line L714 (5.3001, -31.1051) -> (5.2998, -31.1069)
  line L715 (5.2998, -31.1069) -> (5.2989, -31.1085)
  line L716 (5.2989, -31.1085) -> (5.2968, -31.1139)
  line L717 (5.2968, -31.1139) -> (5.2902, -31.1226)
  line L718 (5.2902, -31.1226) -> (5.2845, -31.1318)
  line L719 (5.2845, -31.1318) -> (5.2814, -31.1341)
  line L720 (5.2814, -31.1341) -> (5.279, -31.1371)
  line L721 (5.279, -31.1371) -> (5.2696, -31.1426)
  line L722 (5.2696, -31.1426) -> (5.2608, -31.149)
  line L723 (5.2608, -31.149) -> (5.257, -31.1499)
  line L724 (5.257, -31.1499) -> (5.2537, -31.1518)
  line L725 (5.2537, -31.1518) -> (5.2429, -31.1532)
  line L726 (5.2429, -31.1532) -> (5.2323, -31.1558)
  line L727 (5.2323, -31.1558) -> (5.2285, -31.1552)
  line L728 (5.2285, -31.1552) -> (5.2247, -31.1557)
  line L729 (5.2247, -31.1557) -> (5.2142, -31.1529)
  line L730 (5.2142, -31.1529) -> (5.2034, -31.1511)
  line L731 (5.2034, -31.1511) -> (5.2002, -31.1491)
  line L732 (5.2002, -31.1491) -> (5.1964, -31.1481)
  line L733 (5.1964, -31.1481) -> (5.1878, -31.1415)
  line L734 (5.1878, -31.1415) -> (5.1785, -31.1358)
  line L735 (5.1785, -31.1358) -> (5.1763, -31.1327)
  line L736 (5.1763, -31.1327) -> (5.1732, -31.1303)
  line L737 (5.1732, -31.1303) -> (5.1677, -31.1209)
  line L738 (5.1677, -31.1209) -> (5.1614, -31.1121)
  line L739 (5.1614, -31.1121) -> (5.1595, -31.1066)
  line L740 (5.1595, -31.1066) -> (5.1585, -31.105)
  line L741 (5.1585, -31.105) -> (5.1583, -31.1032)
  line L742 (5.1583, -31.1032) -> (5.1566, -31.0982)
  line L743 (5.1566, -31.0982) -> (4.9185, -30.0982)
  line L744 (4.9185, -30.0982) -> (4.9165, -30.0836)
  line L745 (4.9165, -30.0836) -> (4.9211, -30.0547)
  line L746 (4.9211, -30.0547) -> (4.9365, -30.0298)
  line L747 (4.9365, -30.0298) -> (4.9602, -30.0126)
  line L748 (4.9602, -30.0126) -> (4.9886, -30.0059)
  line L749 (4.9886, -30.0059) -> (5.0175, -30.0105)
  line L750 (5.0175, -30.0105) -> (5.0424, -30.0258)
  line L751 (5.0424, -30.0258) -> (5.0596, -30.0495)
  line L752 (5.0596, -30.0495) -> (5.0644, -30.0634)
  line L753 (5.0644, -30.0634) -> (5.2336, -30.7743)
  line L754 (5.2336, -30.7743) -> (5.3475, -30.3472)
  line L755 (5.3475, -30.3472) -> (5.3488, -30.3438)
  line L756 (5.3488, -30.3438) -> (5.349, -30.3423)
  line L757 (5.349, -30.3423) -> (5.35, -30.3406)
  line L758 (5.35, -30.3406) -> (5.3527, -30.3334)
  line L759 (5.3527, -30.3334) -> (5.3587, -30.3256)
  line L760 (5.3587, -30.3256) -> (5.3637, -30.317)
  line L761 (5.3637, -30.317) -> (5.3675, -30.3141)
  line L762 (5.3675, -30.3141) -> (5.3705, -30.3102)
  line L763 (5.3705, -30.3102) -> (5.379, -30.3052)
  line L764 (5.379, -30.3052) -> (5.3869, -30.2992)
  line L765 (5.3869, -30.2992) -> (5.3916, -30.298)
  line L766 (5.3916, -30.298) -> (5.3958, -30.2955)
  line L767 (5.3958, -30.2955) -> (5.4056, -30.2942)
  line L768 (5.4056, -30.2942) -> (5.4152, -30.2917)
  line L769 (5.4152, -30.2917) -> (5.42, -30.2923)
  line L770 (5.42, -30.2923) -> (5.4248, -30.2917)
  line L771 (5.4248, -30.2917) -> (5.4344, -30.2942)
  line L772 (5.4344, -30.2942) -> (5.4442, -30.2955)
  line L773 (5.4442, -30.2955) -> (5.4484, -30.298)
  line L774 (5.4484, -30.298) -> (5.4531, -30.2992)
  line L775 (5.4531, -30.2992) -> (5.461, -30.3052)
  line L776 (5.461, -30.3052) -> (5.4695, -30.3102)
  line L777 (5.4695, -30.3102) -> (5.4725, -30.3141)
  line L778 (5.4725, -30.3141) -> (5.4763, -30.317)
  line L779 (5.4763, -30.317) -> (5.4813, -30.3256)
  line L780 (5.4813, -30.3256) -> (5.4873, -30.3334)
  line L781 (5.4873, -30.3334) -> (5.49, -30.3406)
  line L782 (5.49, -30.3406) -> (5.491, -30.3423)
  line L783 (5.491, -30.3423) -> (5.4912, -30.3438)
  line L784 (5.4912, -30.3438) -> (5.4925, -30.3472)
  line L785 (5.4925, -30.3472) -> (5.6064, -30.7743)
  line L786 (5.6064, -30.7743) -> (5.7756, -30.0634)
  line L787 (5.7756, -30.0634) -> (5.7804, -30.0495)
  line L788 (5.7804, -30.0495) -> (5.7976, -30.0258)
  line L789 (5.7976, -30.0258) -> (5.8225, -30.0105)
  line L790 (5.8225, -30.0105) -> (5.8514, -30.0059)
  line L791 (5.8514, -30.0059) -> (5.8798, -30.0127)
  line L792 (4.1026, -12.8805) -> (4.1046, -12.8804)
  line L793 (4.1046, -12.8804) -> (4.1072, -12.881)
  line L794 (4.1072, -12.881) -> (4.1099, -12.8813)
  line L795 (4.1099, -12.8813) -> (4.1117, -12.882)
  line L796 (4.1117, -12.882) -> (4.119, -12.8837)
  line L797 (4.119, -12.8837) -> (4.2618, -12.9313)
  line L798 (4.2618, -12.9313) -> (4.2752, -12.9373)
  line L799 (4.2752, -12.9373) -> (4.2973, -12.9565)
  line L800 (4.2973, -12.9565) -> (4.3104, -12.9826)
  line L801 (4.3104, -12.9826) -> (4.3125, -13.0118)
  line L802 (4.3125, -13.0118) -> (4.3033, -13.0396)
  line L803 (4.3033, -13.0396) -> (4.2841, -13.0617)
  line L804 (4.2841, -13.0617) -> (4.2579, -13.0748)
  line L805 (4.2579, -13.0748) -> (4.2287, -13.0768)
  line L806 (4.2287, -13.0768) -> (4.2144, -13.0736)
  line L807 (4.2144, -13.0736) -> (4.0831, -13.0298)
  line L808 (4.0831, -13.0298) -> (3.8748, -13.0298)
  line L809 (3.8748, -13.0298) -> (3.8063, -13.0641)
  line L810 (3.8063, -13.0641) -> (3.7759, -13.0945)
  line L811 (3.7759, -13.0945) -> (3.7417, -13.163)
  line L812 (3.7417, -13.163) -> (3.7417, -13.2228)
  line L813 (3.7417, -13.2228) -> (3.7759, -13.2913)
  line L814 (3.7759, -13.2913) -> (3.8063, -13.3218)
  line L815 (3.8063, -13.3218) -> (3.8833, -13.3602)
  line L816 (3.8833, -13.3602) -> (4.0658, -13.4059)
  line L817 (4.0658, -13.4059) -> (4.0669, -13.4063)
  line L818 (4.0669, -13.4063) -> (4.0674, -13.4063)
  line L819 (4.0674, -13.4063) -> (4.0735, -13.4086)
  line L820 (4.0735, -13.4086) -> (4.0797, -13.4108)
  line L821 (4.0797, -13.4108) -> (4.0801, -13.4111)
  line L822 (4.0801, -13.4111) -> (4.0812, -13.4115)
  line L823 (4.0812, -13.4115) -> (4.1764, -13.4592)
  line L824 (4.1764, -13.4592) -> (4.1827, -13.4631)
  line L825 (4.1827, -13.4631) -> (4.1845, -13.4639)
  line L826 (4.1845, -13.4639) -> (4.1866, -13.4656)
  line L827 (4.1866, -13.4656) -> (4.1888, -13.467)
  line L828 (4.1888, -13.467) -> (4.1901, -13.4685)
  line L829 (4.1901, -13.4685) -> (4.1959, -13.4732)
  line L830 (4.1959, -13.4732) -> (4.2435, -13.5208)
  line L831 (4.2435, -13.5208) -> (4.2482, -13.5266)
  line L832 (4.2482, -13.5266) -> (4.2497, -13.5279)
  line L833 (4.2497, -13.5279) -> (4.2511, -13.5301)
  line L834 (4.2511, -13.5301) -> (4.2528, -13.5322)
  line L835 (4.2528, -13.5322) -> (4.2536, -13.534)
  line L836 (4.2536, -13.534) -> (4.2576, -13.5403)
  line L837 (4.2576, -13.5403) -> (4.3052, -13.6356)
  line L838 (4.3052, -13.6356) -> (4.3104, -13.6493)
  line L839 (4.3104, -13.6493) -> (4.3106, -13.652)
  line L840 (4.3106, -13.652) -> (4.3117, -13.6545)
  line L841 (4.3117, -13.6545) -> (4.3131, -13.6691)
  line L842 (4.3131, -13.6691) -> (4.3131, -13.7643)
  line L843 (4.3131, -13.7643) -> (4.3117, -13.779)
  line L844 (4.3117, -13.779) -> (4.3106, -13.7815)
  line L845 (4.3106, -13.7815) -> (4.3104, -13.7842)
  line L846 (4.3104, -13.7842) -> (4.3052, -13.7979)
  line L847 (4.3052, -13.7979) -> (4.2576, -13.8931)
  line L848 (4.2576, -13.8931) -> (4.2536, -13.8994)
  line L849 (4.2536, -13.8994) -> (4.2528, -13.9012)
  line L850 (4.2528, -13.9012) -> (4.2511, -13.9033)
  line L851 (4.2511, -13.9033) -> (4.2497, -13.9056)
  line L852 (4.2497, -13.9056) -> (4.2482, -13.9069)
  line L853 (4.2482, -13.9069) -> (4.2435, -13.9126)
  line L854 (4.2435, -13.9126) -> (4.1959, -13.9602)
  line L855 (4.1959, -13.9602) -> (4.1901, -13.9649)
  line L856 (4.1901, -13.9649) -> (4.1888, -13.9664)
  line L857 (4.1888, -13.9664) -> (4.1866, -13.9679)
  line L858 (4.1866, -13.9679) -> (4.1845, -13.9696)
  line L859 (4.1845, -13.9696) -> (4.1827, -13.9703)
  line L860 (4.1827, -13.9703) -> (4.1764, -13.9743)
  line L861 (4.1764, -13.9743) -> (4.0812, -14.0219)
  line L862 (4.0812, -14.0219) -> (4.0674, -14.0272)
  line L863 (4.0674, -14.0272) -> (4.0647, -14.0273)
  line L864 (4.0647, -14.0273) -> (4.0623, -14.0284)
  line L865 (4.0623, -14.0284) -> (4.0476, -14.0298)
  line L866 (4.0476, -14.0298) -> (3.8095, -14.0298)
  line L867 (3.8095, -14.0298) -> (3.8021, -14.0291)
  line L868 (3.8021, -14.0291) -> (3.8001, -14.0292)
  line L869 (3.8001, -14.0292) -> (3.7975, -14.0286)
  line L870 (3.7975, -14.0286) -> (3.7949, -14.0284)
  line L871 (3.7949, -14.0284) -> (3.7931, -14.0276)
  line L872 (3.7931, -14.0276) -> (3.7858, -14.026)
  line L873 (3.7858, -14.026) -> (3.6429, -13.9784)
  line L874 (3.6429, -13.9784) -> (3.6295, -13.9724)
  line L875 (3.6295, -13.9724) -> (3.6074, -13.9532)
  line L876 (3.6074, -13.9532) -> (3.5943, -13.927)
  line L877 (3.5943, -13.927) -> (3.5923, -13.8978)
  line L878 (3.5923, -13.8978) -> (3.6015, -13.8701)
  line L879 (3.6015, -13.8701) -> (3.6207, -13.848)
  line L880 (3.6207, -13.848) -> (3.6469, -13.8349)
  line L881 (3.6469, -13.8349) -> (3.676, -13.8328)
  line L882 (3.676, -13.8328) -> (3.6904, -13.836)
  line L883 (3.6904, -13.836) -> (3.8217, -13.8798)